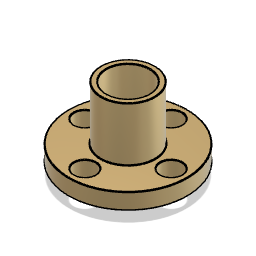
table skilllll v16 (Autodesk Fusion 360 archive; units mm, degrees)
design "Leadscrew Nut"
Autodesk Fusion 360 part; units mm, degrees
sketch "Sketch1" plane through (0, 0, 0) normal (0, 1, 0) x (1, 0, 0)
  circle A0 centre (0, 0) radius 5
  circle A1 centre (0, 0) radius 11
  circle A2 centre (0, 0) radius 4
  circle A3 centre (8, 0) radius 2
  circle A4 centre (0, 8) radius 2
  circle A5 centre (-8, 0) radius 2
  circle A6 centre (0, -8) radius 2
  dimension "d1" = 10
  dimension "d8" = 22
  dimension "d11" = 8
  dimension "d15" = 4
  dimension "d17" = 4
  dimension "d18" = 4
  dimension "d19" = 4
  constraint coincident A0.centre A1.centre
  constraint concentric A0 A1
  constraint concentric A1 A2
  measures "d1" diameter of A0
  measures "d8" diameter of A1
  measures "d11" diameter of A2
  measures "d15" diameter of A3
  measures "d17" diameter of A4
  measures "d18" diameter of A5
  measures "d19" diameter of A6
sketch "Sketch2" plane through (0, 0, 0) normal (0, 1, 0) x (1, 0, 0)
  line L0 (-25, 25) -> (25, 25)
  line L1 (25, 25) -> (25, -25)
  line L2 (25, -25) -> (-25, -25)
  line L3 (-25, -25) -> (-25, 25)
  constraint horizontal L0
  constraint vertical L1
  constraint horizontal L2
  constraint vertical L3
extrude "Extrude1" add sketch "Sketch1" along normal blind 3 contours A0 | A1 in component "Component"
extrude "Extrude2" add sketch "Sketch1" along normal blind 13 and the other way blind 2 contours A0 in component "Component"
chamfer "Chamfer1" distance 0.1 angle 45 16 edges at (-9.8647, 3, -0.7232) (-3.7293, 13, -1.4465) (-4.6616, 3, -1.8081) (6.1353, 3, -0.7232) (-1.8647, 3, -8.7232) (-1.8647, 3, 7.2768) (-4.6616, -2, -1.8081) (-10.2556, 0, 3.9778) (-4.6616, 13, 1.8081) (6.1353, 0, -0.7232) (-9.8647, 0, -0.7232) (-10.2556, 3, 3.9778) (-1.8647, 0, 7.2768) (-3.7293, -2, 1.4465) (-4.6616, 0, 1.8081) (-1.8647, 0, -8.7232) in component "Component"
component "Component" placed x (1, 0, 0) y (0, 1, 0) z (0, 0, 1) at (0, 0, 0)
